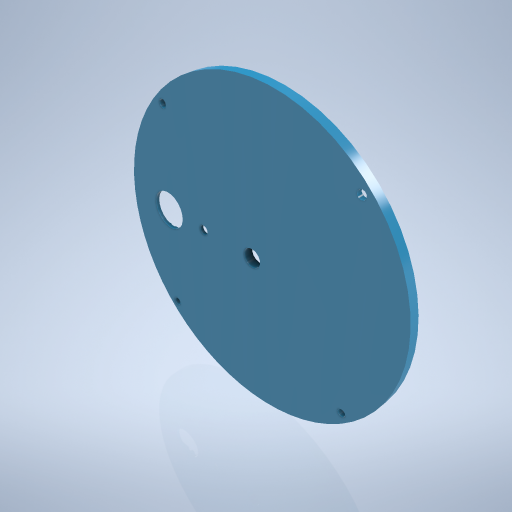
# Autodesk Inventor part: plate_2
Saved by Autodesk Inventor 2024.2 (Build 282272000, 272)
## iProperties
Created: 2024-04-01
Part Number: plate_2
Material: Gold
Document SubType Name: Modeling
Designer: Fabri
Density: 19.3 g/cm^3
Appearance: Himmelblau - dunkel
Author: Fabri
Autodesk Inventor part; units mm, degrees
note: some values were not read from the file. Chosen so that the rebuilt part matches the saved one: direction of "Bohrung3"; direction of "Bohrung4"; direction of "Bohrung5"; direction of "Bohrung6".
ref_plane "YZ Plane" through (0, 0, 0) normal (1, 0, 0) x (0, 1, 0)
ref_plane "XZ Plane" through (0, 0, 0) normal (0, 1, 0) x (-1, 0, 0)
sketch "Skizze1" plane through (0, 0, 0) normal (0, 0, 1) x (1, 0, 0)
  line L0 (0, 0) -> (0, 15)
  line L1 (0, 3) -> (-9, 3)
  line L2 (-9, 3) -> (-9.567, 2.0179)
  arc A0 (-10.433, 2.0179) -> (-9.567, 2.0179) centre (-10, 2.2679) ccw
  line L3 (-10.433, 2.0179) -> (-11, 3)
  line L4 (-11, 3) -> (-12, 3)
  line L5 (-12, 3) -> (-12.567, 2.0179)
  arc A1 (-13.433, 2.0179) -> (-12.567, 2.0179) centre (-13, 2.2679) ccw
  line L6 (-13.433, 2.0179) -> (-14, 3)
  line L7 (-10, 2.2679) -> (-10, 5.291) construction
  line L8 (-14, 3) -> (-15, 3)
  line L9 (-15, 3) -> (-15.567, 2.0179)
  arc A2 (-16.433, 2.0179) -> (-15.567, 2.0179) centre (-16, 2.2679) ccw
  line L10 (-16.433, 2.0179) -> (-17, 3)
  line L11 (-17, 3) -> (-18, 3)
  line L12 (-18, 3) -> (-18.567, 2.0179)
  arc A3 (-19.433, 2.0179) -> (-18.567, 2.0179) centre (-19, 2.2679) ccw
  line L13 (-19.433, 2.0179) -> (-20, 3)
  line L14 (-20, 3) -> (-21, 3)
  line L15 (-21, 3) -> (-21.567, 2.0179)
  arc A4 (-22.433, 2.0179) -> (-21.567, 2.0179) centre (-22, 2.2679) ccw
  line L16 (-22.433, 2.0179) -> (-23, 3)
  line L17 (-23, 3) -> (-24, 3)
  line L18 (-24, 3) -> (-24.567, 2.0179)
  arc A5 (-25.433, 2.0179) -> (-24.567, 2.0179) centre (-25, 2.2679) ccw
  line L19 (-25.433, 2.0179) -> (-26, 3)
  line L20 (-26, 3) -> (-27, 3)
  line L21 (-27, 3) -> (-27.567, 2.0179)
  arc A6 (-28.433, 2.0179) -> (-27.567, 2.0179) centre (-28, 2.2679) ccw
  line L22 (-28.433, 2.0179) -> (-29, 3)
  line L23 (-29, 3) -> (-30, 3)
  line L24 (-30, 3) -> (-30.567, 2.0179)
  arc A7 (-31.433, 2.0179) -> (-30.567, 2.0179) centre (-31, 2.2679) ccw
  line L25 (-31.433, 2.0179) -> (-32, 3)
  line L26 (-32, 3) -> (-33, 3)
  line L27 (-33, 3) -> (-33.567, 2.0179)
  arc A8 (-34.433, 2.0179) -> (-33.567, 2.0179) centre (-34, 2.2679) ccw
  line L28 (-34.433, 2.0179) -> (-35, 3)
  line L29 (-35, 3) -> (-36, 3)
  line L30 (-36, 3) -> (-36.567, 2.0179)
  arc A9 (-37.433, 2.0179) -> (-36.567, 2.0179) centre (-37, 2.2679) ccw
  line L31 (-37.433, 2.0179) -> (-38, 3)
  line L32 (-38, 3) -> (-50, 3)
  line L33 (-50, 3) -> (-50, 0)
  line L34 (-50, 0) -> (0, 0)
  line L35 (0, 3) -> (0, 0)
  dimension "d0" = 15
  dimension "d2" = 60
  dimension "d3" = 3
  dimension "d4" = 2
  dimension "d7" = 3
  dimension "d12" = 3
  dimension "d13" = 100
  dimension "d14" = 20
  dimension "d50" = 0.5
  constraints: 72 end point, 20 point on circle, 10 centre point, 10 point on line, 4 tangent, 3 horizontal, 3 horizontal alignment, 3 parallel, 3 perpendicular, 2 vertical, 1 collinear, 1 equal radius, 1 symmetric about line, 80 other
  measures "d0" distance of L0.start L0.end
  measures "d2" angle of L2 L3
  measures "d3" distance of A1.centre L7.start
  measures "d4" distance of L4.end L6.end
  measures "d7" distance of L3.end L8.start
  measures "d12" distance of L32.end L33.end
  measures "d13" diameter of L33 L0
  measures "d14" diameter of L7.start L0
  measures "d50" radius of A0
revolve "Umdrehung1" add sketch "Skizze1" angle 360 about axis through (0, 0, 0) along (0, 1, 0)
ref_plane "Arbeitsebene1" through (0, 1.2, 0) normal (0, 1, 0) x (1, 0, 0)
sketch "Skizze7" plane through (0, 1.2, 0) normal (0, 1, 0) x (1, 0, 0)
  line L0 (0, 0) -> (-82.9092, 0) construction
  circle A0 centre (0, 0) radius 50 projected
  line L1 (-11.8, -7.5) -> (-49.4343, -7.5)
  line L2 (-49.4343, 7.5) -> (-11.8, 7.5)
  line L3 (-11.8, 7.5) -> (-11.8, -7.5)
  dimension "d58" = 11.8
  dimension "d59" = 15
  constraints: 8 end point, 2 horizontal, 2 point on circle, 1 parallel, 1 symmetric about line, 1 other
  measures "d58" distance from line of L3 L0.start
  measures "d59" distance between parallel lines of L2 L1
extrude "Extrusion3" cut sketch "Skizze7" along normal up to surface (1.8 mm away) contours L2 L3 L1 A0 picked at (-24.5123, -0.8361)
fillet "Rundung1" radius 2 2 edges at (-11.8, 2.0842, -7.5) (-11.8, 2.0842, 7.5)
sketch "Skizze6" plane through (0, 3, 0) normal (0, 1, 0) x (1, 0, 0)
  circle A0 centre (0, 0) radius 9 projected
  constraints: 1 coincident
hole "Bohrung3" at (0, 3, 0) direction (0, -1, 0) diameter 6 depth 3
sketch "Skizze8" plane through (-49.4343, 3, -7.5) normal (0, 1, 0) x (1, 0, 0)
  arc A0 (37.5119, -13.6889) -> (37.5119, -1.3111) centre (49.4343, -7.5) ccw projected
  line L0 (49.4343, -7.5) -> (49.4343, -67.1746) construction
  circle A1 centre (49.4343, -7.5) radius 3 projected
  line L1 (49.4343, -7.5) -> (3.1855, -53.7488) construction
  point P0 (16.2003, -40.734)
  point P1 (38.29, -15)
  point P2 (38.29, 0)
  dimension "d70" = 45
  dimension "d71" = 47
  constraints: 4 end point, 1 point on line, 1 vertical
  measures "d70" angle of L1 L0
  measures "d71" distance of point (49.434, -7.5) point (16.2, -40.734)
hole "Bohrung4" at (-33.234, 3, 33.234) direction (0, -1, 0) diameter 2.7 depth 3 countersink diameter 5.5 countersink angle 90
pattern_circular "Runde Anordnung2" count 4 over 360 about axis through (0, 1.5, 0) along (0, 1, 0) of "Bohrung4"
sketch "Skizze9" plane through (0, 1.2, 0) normal (0, 1, 0) x (1, 0, 0)
  point P0 (0, 0)
  point P1 (-34, 0)
  dimension "d82" = 34
  constraints: 1 horizontal alignment
  measures "d82" distance of point (-34, 0) point (0, 0)
hole "Bohrung5" at (-34, 1.2, 0) direction (0, -1, 0) diameter 12 depth 1.2
sketch "Skizze10" plane through (0, 1.2, 0) normal (0, 1, 0) x (1, 0, 0)
  point P0 (0, 0)
  point P1 (-19, 0)
  dimension "d90" = 19
  constraints: 1 horizontal alignment
  measures "d90" distance of point (-19, 0) point (0, 0)
hole "Bohrung6" at (-19, 1.2, 0) direction (0, -1, 0) diameter 3.2 depth 1.2
